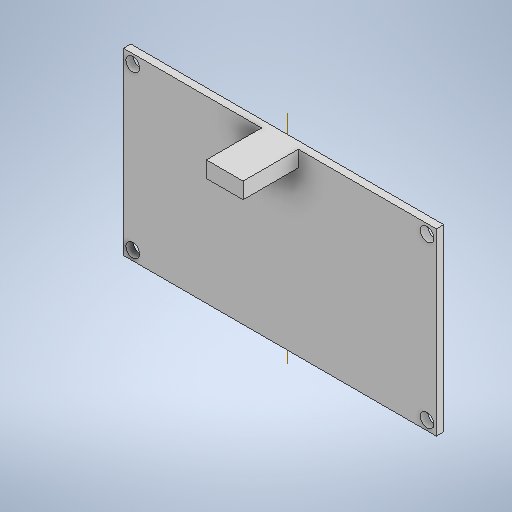
# Autodesk Inventor part: 컨버터
Saved by Autodesk Inventor 2025 (Build 290162000, 162)
## iProperties
Created: 2024-06-01
Part Number: 컨버터
Material: 일반
Document SubType Name: Modeling
Designer: ckhye
Density: 1 g/cm^3
Appearance: 기본값
Author: ckhye
Autodesk Inventor part; units mm, degrees
ref_plane "YZ Plane" through (0, 0, 0) normal (1, 0, 0) x (0, 1, 0)
ref_plane "XZ Plane" through (0, 0, 0) normal (0, 1, 0) x (-1, 0, 0)
ref_plane "XY Plane" through (0, 0, 0) normal (0, 0, 1) x (1, 0, 0)
sketch "스케치1" plane through (0, 0, 0) normal (0, 0, 1) x (1, 0, 0)
  line L0 (-34, 19.5) -> (34, 19.5)
  line L1 (34, 19.5) -> (34, -19.5)
  line L2 (34, -19.5) -> (-34, -19.5)
  line L3 (-34, -19.5) -> (-34, 19.5)
  line L4 (-34, 19.5) -> (34, -19.5) construction
  line L5 (34, 19.5) -> (-34, -19.5) construction
  point P0 (0, 0)
  dimension "d0" = 68
  dimension "d1" = 39
  constraints: 12 end point, 2 midpoint, 2 parallel, 1 horizontal, 1 perpendicular
  measures "d0" distance of L1.end L2.end
  measures "d1" distance between parallel lines of L2 L0
extrude "돌출1" add sketch "스케치1" along normal blind 1.6
sketch "스케치3" plane through (0, 0, 1.6) normal (0, 0, 1) x (1, 0, 0)
  circle A0 centre (32, 17.5) radius 2
  circle A1 centre (-32, 17.5) radius 2
  circle A2 centre (-32, -17.5) radius 2
  circle A3 centre (32, -17.5) radius 2
  line L0 (34, 19.5) -> (-34, 19.5) projected
  line L1 (34, -19.5) -> (34, 19.5) projected
  line L2 (-34, -19.5) -> (34, -19.5) projected
  line L3 (-34, 19.5) -> (-34, -19.5) projected
  circle A4 centre (-32, 17.5) radius 1.5
  circle A5 centre (32, 17.5) radius 1.5
  circle A6 centre (32, -17.5) radius 1.5
  circle A7 centre (-32, -17.5) radius 1.5
  point P0 (0, 0)
  dimension "d4" = 4
  dimension "d5" = 4
  dimension "d6" = 4
  dimension "d7" = 4
  dimension "d8" = 3
  dimension "d9" = 3
  dimension "d10" = 3
  dimension "d11" = 3
  constraints: 8 centre point, 8 tangent, 4 coincident
  measures "d4" diameter of A0
  measures "d5" diameter of A1
  measures "d6" diameter of A2
  measures "d7" diameter of A3
  measures "d8" diameter of A4
  measures "d9" diameter of A5
  measures "d10" diameter of A6
  measures "d11" diameter of A7
extrude "돌출2" cut sketch "스케치3" against normal up to surface (1.6 mm away) contours A4 | A5 | A6 | A7
sketch "스케치4" plane through (0, 0, 1.6) normal (0, 0, 1) x (1, 0, 0)
  line L0 (4, 15.9921) -> (-4, 15.9921)
  line L1 (-4, 15.9921) -> (-4, 19.5)
  line L2 (-4, 19.5) -> (4, 19.5)
  line L3 (4, 19.5) -> (4, 15.9921)
  line L4 (4, 15.9921) -> (-4, 19.5) construction
  line L5 (-4, 15.9921) -> (4, 19.5) construction
  line L6 (34, 19.5) -> (-34, 19.5) projected
  line L7 (0, -27.3) -> (0, 27.3) projected
  point P0 (0, 0)
  point P1 (0, 17.746)
  point P2 (0, 19.5)
  point P3 (-4, 17.746)
  dimension "d14" = 8
  constraints: 12 end point, 5 midpoint, 2 parallel, 1 horizontal, 1 perpendicular, 1 point on line
  measures "d14" distance from line of point (-4, 17.746) L3
extrude "돌출3" add sketch "스케치4" along normal blind 12
